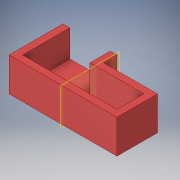
# Autodesk Inventor part: hookSupport
Saved by Autodesk Inventor 2018.2 (Build 222227000, 227)
## iProperties
Created: 2018-03-20
Part Number: hookSupport
Material: PBT Plastic
Document SubType Name: Modeling
Designer: steele
Density: 1.31 g/cm^3
Appearance: Smooth - Red
Author: steele
Autodesk Inventor part; units mm, degrees
ref_plane "XZ Plane" through (0, 0, 0) normal (0, 1, 0) x (-1, 0, 0)
ref_plane "XY Plane" through (0, 0, 0) normal (0, 0, 1) x (1, 0, 0)
sketch "Sketch1" plane through (0, 0, 0) normal (0, 0, 1) x (1, 0, 0)
  line L0 (-50.8, -15.875) -> (50.8, -15.875)
  line L1 (50.8, -15.875) -> (50.8, 15.875)
  line L2 (50.8, 15.875) -> (-50.8, 15.875)
  line L3 (-50.8, 15.875) -> (-50.8, -15.875)
  line L4 (-50.8, -15.875) -> (50.8, 15.875) construction
  line L5 (50.8, -15.875) -> (-50.8, 15.875) construction
  point P0 (0, 0)
  dimension "d0" = 101.6
  dimension "d1" = 31.75
  constraints: 12 end point, 2 midpoint, 2 parallel, 1 horizontal, 1 perpendicular
  measures "d0" distance of L1.end L2.end
  measures "d1" distance of L2.end L0.start
extrude "Extrusion1" add sketch "Sketch1" along normal mid plane 38.1
sketch "Sketch3" plane through (-50.8, 15.875, 19.05) normal (0, 1, 0) x (1, 0, 0)
  line L0 (95.25, 6.35) -> (95.25, 31.75)
  line L1 (95.25, 31.75) -> (6.35, 31.75)
  line L2 (6.35, 31.75) -> (6.35, 6.35)
  line L3 (6.35, 6.35) -> (95.25, 6.35)
  line L4 (95.25, 6.35) -> (6.35, 31.75) construction
  line L5 (95.25, 31.75) -> (6.35, 6.35) construction
  line L6 (0, 38.1) -> (0, 0) projected
  line L7 (0, 38.1) -> (101.6, 38.1) projected
  point P0 (50.8, 19.05)
  dimension "d4" = 6.35
  dimension "d5" = 6.35
  constraints: 12 end point, 2 midpoint, 2 parallel, 1 perpendicular, 1 vertical
  measures "d4" distance between parallel lines of L6 L2
  measures "d5" distance between parallel lines of L7 L1
extrude "Extrusion2" cut sketch "Sketch3" against normal blind 25.4
sketch "Sketch8" plane through (-44.45, 15.875, -12.7) normal (0, 0, 1) x (1, 0, 0)
  line L0 (88.9, 0) -> (0, 0) projected
  line L1 (0, 0) -> (38.1, 0)
  line L2 (38.1, 0) -> (38.1, -25.4)
  line L3 (38.1, -25.4) -> (0, -25.4)
  line L4 (0, -25.4) -> (0, 0)
  point P0 (44.45, -15.875)
  dimension "d14" = 38.1
  dimension "d15" = 25.4
  constraints: 8 end point, 2 parallel, 1 horizontal, 1 perpendicular
  measures "d14" distance of L2.end L3.end
  measures "d15" distance of L1.end L2.end
extrude "Extrusion5" cut sketch "Sketch8" against normal through all
sketch "Sketch9" plane through (0, 0, -19.05) normal (0, 0, -1) x (-1, 0, 0)
  line L0 (50.8, -15.875) -> (50.8, 15.875) projected
  line L1 (50.8, 15.875) -> (50.8, -15.875)
  line L2 (50.8, -15.875) -> (0, -15.875)
  line L3 (-50.8, -15.875) -> (50.8, -15.875) projected
  line L4 (0, -15.875) -> (0, 15.875)
  line L5 (-50.8, 15.875) -> (50.8, 15.875) projected
  line L6 (6.35, -9.525) -> (6.35, 15.875) projected
  line L7 (6.35, 15.875) -> (6.35, -9.525)
  line L8 (44.45, 15.875) -> (44.45, -9.525) projected
  line L9 (6.35, -9.525) -> (44.45, -9.525)
  line L10 (44.45, -9.525) -> (44.45, 15.875)
  line L11 (44.45, 15.875) -> (50.8, 15.875)
  point P0 (0, 0)
  dimension "d18" = 50.8
  constraints: 14 end point, 3 collinear, 2 midpoint, 2 perpendicular
  measures "d18" distance of L0.start L2.end
extrude "Extrusion6" add sketch "Sketch9" along normal blind 12.7 contours L2 L4 L5 L6 L9 L8 L0
body "Solid1"
